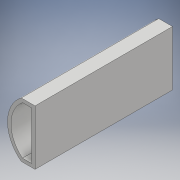
# Autodesk Inventor part: Sanding Block
Saved by Autodesk Inventor 2018.1 (Build 221171000, 171)
## iProperties
Created: 2017-10-26
Part Number: Sanding Block
Material: Generic
Document SubType Name: Modeling
Designer: xdlea
Density: 1 g/cm^3
Appearance: Default
Author: xdlea
Autodesk Inventor part; units mm, degrees
ref_plane "YZ Plane" through (0, 0, 0) normal (1, 0, 0) x (0, 1, 0)
ref_plane "XZ Plane" through (0, 0, 0) normal (0, 1, 0) x (-1, 0, 0)
ref_plane "XY Plane" through (0, 0, 0) normal (0, 0, 1) x (1, 0, 0)
sketch "Sketch1" plane through (0, 0, 0) normal (0, 1, 0) x (-1, 0, 0)
  line L0 (-5, 20) -> (5, 20)
  line L1 (5, 20) -> (5, -20) construction
  line L2 (5, -20) -> (-5, -20)
  line L3 (-5, -20) -> (-5, 20)
  line L4 (-5, 20) -> (5, -20) construction
  line L5 (5, 20) -> (-5, -20) construction
  arc A0 (5, -20) -> (5, 20) centre (-10, 0) ccw
  line L6 (-2.5, -17.5) -> (4.1421, -17.5)
  arc A1 (4.1421, -17.5) -> (4.1421, 17.5) centre (-10, 0) ccw
  line L7 (4.1421, 17.5) -> (-2.5, 17.5)
  line L8 (-2.5, 17.5) -> (-2.5, -17.5)
  point P0 (0, 0)
  dimension "d0" = 25
  dimension "d1" = 10
  dimension "d3" = 40
  dimension "d7" = 2.5
  constraints: 18 end point, 4 point on circle, 3 parallel, 2 centre point, 2 midpoint, 1 horizontal, 1 perpendicular, 3 other
  measures "d0" radius of A0
  measures "d1" distance of L1.end L2.end
  measures "d3" distance of L2.end L0.start
  measures "d7" radial gap between concentric circles of A0 A1
extrude "Extrusion1" add sketch "Sketch1" along normal blind 100
body "Solid1"
